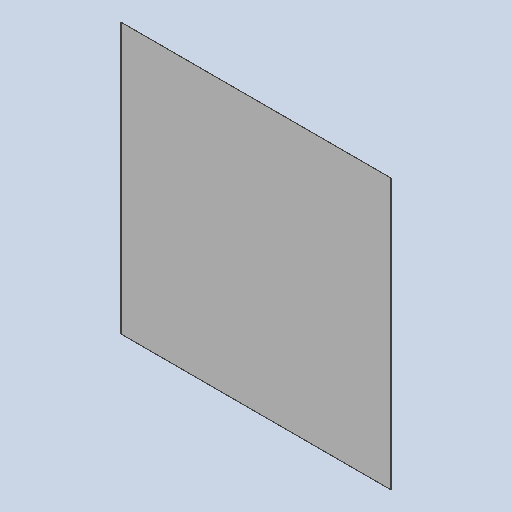
# Autodesk Inventor part: Boden
Saved by Autodesk Inventor 2025.1 (Build 291241000, 241)
## iProperties
Created: 2024-10-13
Part Number: Boden
Material: Generisch
Document SubType Name: Modeling
Designer: Kai Altwicker
Density: 1 g/cm^3
Appearance: Vorgabe
Mass: 2.25e+06 g
Surface Area: 4.506e+06 cm^2
Volume: 2.25e+06 cm^3
Author: Kai Altwicker
Autodesk Inventor part; units mm, degrees
ref_plane "YZ Plane" through (0, 0, 0) normal (1, 0, 0) x (0, 1, 0)
ref_plane "XZ Plane" through (0, 0, 0) normal (0, 1, 0) x (-1, 0, 0)
ref_plane "XY Plane" through (0, 0, 0) normal (0, 0, 1) x (1, 0, 0)
ref_plane "Arbeitsebene1" through (0, 0, 0) normal (0, 0, 1) x (1, 0, 0)
sketch "Skizze1" plane through (0, 0, 0) normal (0, 0, 1) x (1, 0, 0)
  line L0 (7500, -7500) -> (-7500, -7500)
  line L1 (-7500, -7500) -> (-7500, 7500)
  line L2 (-7500, 7500) -> (7500, 7500)
  line L3 (7500, 7500) -> (7500, -7500)
  point P0 (0, 0)
  point P1 (-7500, 0)
  point P2 (0, 7500)
  dimension "d0" = 15000
  constraints: 8 end point, 2 midpoint, 2 parallel, 2 perpendicular, 1 horizontal, 1 horizontal alignment, 1 vertical alignment
  measures "d0" distance of L0.end L1.end
extrude "Extrusion1" add sketch "Skizze1" against normal blind 10
equation "\"d_tol\" = 0.3"
equation "\"d_wand\" = 1.5"
equation "\"D_oct\" = 3621.32034"
equation "\"d_traeger\" = 625"
